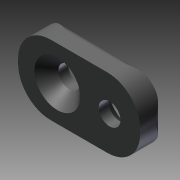
# Autodesk Inventor part: UWANGFplate
Saved by Autodesk Inventor 2011 SP1 (Build 150282100, 282)
## iProperties
Created: 2015-02-05
Part Number: UWANGFplate
Catalog Web Link: www.cadenas.de
Description: UWANGF, UWANSGF_plate-Pulls with Plates - Plate
Vendor: MISUMI
Document SubType Name: Modeling
Designer: psAdmin
Manufacturer: MISUMI
Mass: 1.61867 g
Surface Area: 11.9145 cm^2
Volume: 1.61867 cm^3
Density: 1 g/cm^3
Category: PARTsolutions
Company: MISUMI
Title: UWANGFplate
Author: Cadenas PARTsolutions
Comments: Pulls with Plates - Plate
PSOL_IDENT_0: {\\10.0.0.236\data_v8\23d-libs\misumi\metric\39_accessories_for_al_extrusions\uwangf_plate.prj},179
PSOL_IDENT_1: {VTYP=3D},{NB=UWANGFplate},{LINA=UWANGFplate},{NN=UWANGF, UWANSGF_plate},{DATE=17.11.2014 05:31:37},
PSOL_IDENT_2: {GEOMDATE=19.02.2010 07:36:00},{VERSION=},{LINEID=10},{LINESUBID=-1},{WBVAR=}  {NB=UWANGFplate},{LIN
PSOL_IDENT_3: A=UWANGFplate},{KT=DUMMY},{PN=UWANGFplate}
SUPPLIER: MISUMI
ARTICLENO: UWANGFplate
BOMINFO: UWANGFplate
CREATOR: CADENAS GmbH
Autodesk Inventor part; units mm, degrees
ref_plane "YZ Plane" through (0, 0, 0) normal (1, 0, 0) x (0, 1, 0)
ref_plane "XZ Plane" through (0, 0, 0) normal (0, 1, 0) x (-1, 0, 0)
ref_plane "XY Plane" through (0, 0, 0) normal (0, 0, 1) x (1, 0, 0)
sketch "Sketch_1" plane through (0, 0, 0) normal (0, 0, 1) x (1, 0, 0)
  line L0 (0, 0) -> (28, 0)
  line L1 (28, 0) -> (28, 3.5)
  arc A0 (28, 3.5) -> (26.5, 5) centre (26.5, 3.5) ccw
  line L2 (26.5, 5) -> (1.5, 5)
  arc A1 (1.5, 5) -> (0, 3.5) centre (1.5, 3.5) ccw
  line L3 (0, 3.5) -> (0, 0)
  constraints: 8 end point, 4 point on circle, 2 centre point
extrude "Extrusion1" add sketch "Sketch_1" along normal mid plane 16
sketch "Sketch_2" plane through (0, 0, 0) normal (1, 0, 0) x (0, 1, 0)
  line L0 (14.3017, 20.7284) -> (-9.9569, 20.7284)
  line L1 (-9.9569, 20.7284) -> (-9.9569, -18.375)
  line L2 (-9.9569, -18.375) -> (14.3017, -18.375)
  line L3 (14.3017, -18.375) -> (14.3017, 20.7284)
  line L4 (0, 8) -> (0, -8)
  line L5 (0, -8) -> (3.5, -8)
  arc A0 (3.5, -8) -> (5, -6.5) centre (3.5, -6.5) ccw
  line L6 (5, -6.5) -> (5, 6.5)
  arc A1 (5, 6.5) -> (3.5, 8) centre (3.5, 6.5) ccw
  line L7 (3.5, 8) -> (0, 8)
  constraints: 16 end point, 4 point on circle, 2 centre point
extrude "Extrusion2" cut sketch "Sketch_2" along normal blind 28
sketch "Sketch_3" plane through (0, 0, 0) normal (0, 0, 1) x (1, 0, 0)
  line L0 (21, 0) -> (21, 5)
  line L1 (21, 5) -> (26.25, 5)
  line L2 (26.25, 5) -> (23.5, 2.25)
  line L3 (23.5, 2.25) -> (23.5, 0)
  line L4 (23.5, 0) -> (21, 0)
  line L5 (21, 0) -> (21, 5)
  constraints: 12 end point
revolve "Revolution1" cut sketch "Sketch_3" angle 360 about axis through (21, 0, 0) along (0, -1, 0)
sketch "Sketch_4" plane through (0, 0, 0) normal (0, 0, 1) x (1, 0, 0)
  line L0 (9, 0) -> (9, 5)
  line L1 (9, 5) -> (11.5, 5)
  line L2 (11.5, 5) -> (11.5, 2.75)
  line L3 (11.5, 2.75) -> (14.25, 0)
  line L4 (14.25, 0) -> (9, 0)
  line L5 (9, 0) -> (9, 5)
  constraints: 12 end point
revolve "Revolution2" cut sketch "Sketch_4" angle 360 about axis through (9, 0, 0) along (0, -1, 0)
sketch "Sketch_7" plane through (0, 0, 0) normal (0, 1, 0) x (-1, 0, 0)
  line L0 (14, -16) -> (14, 16)
  line L1 (14, 16) -> (-34, 16)
  line L2 (-34, 16) -> (-34, -16)
  line L3 (-34, -16) -> (14, -16)
  arc A0 (0, 0.5) -> (-7.5, 8) centre (-7.5, 0.5) ccw
  line L4 (-7.5, 8) -> (-20.5, 8)
  arc A1 (-20.5, 8) -> (-28, 0.5) centre (-20.5, 0.5) ccw
  line L5 (-28, 0.5) -> (-28, -0.5)
  arc A2 (-28, -0.5) -> (-20.5, -8) centre (-20.5, -0.5) ccw
  line L6 (-20.5, -8) -> (-7.5, -8)
  arc A3 (-7.5, -8) -> (0, -0.5) centre (-7.5, -0.5) ccw
  line L7 (0, -0.5) -> (0, 0.5)
  constraints: 16 end point, 8 point on circle, 4 centre point
extrude "Extrusion3" cut sketch "Sketch_7" along normal blind 5
ref_plane "frame_bolt_XY" through (21, 2.25, 0) normal (0, 1, 0) x (1, 0, 0)
ref_plane "frame_bolt_YZ" through (21, 2.25, 0) normal (1, 0, 0) x (0, 0, -1)
ref_plane "frame_bolt_ZX" through (21, 2.25, 0) normal (0, 0, -1) x (0, 1, 0)
ref_plane "pull_bolt_XY" through (9, 2.75, 0) normal (0, -1, 0) x (1, 0, 0)
ref_plane "pull_bolt_YZ" through (9, 2.75, 0) normal (1, 0, 0) x (0, 0, 1)
ref_plane "pull_bolt_ZX" through (9, 2.75, 0) normal (0, 0, 1) x (0, -1, 0)
body "Solid1"
